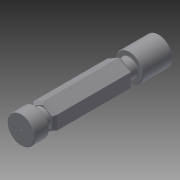
# Autodesk Inventor part: Part1
Saved by Autodesk Inventor 2015 SP2 (Build 190223200, 223)
## iProperties
Created: 2015-11-09
Part Number: Part1
Material: Generic
Document SubType Name: Modeling
Designer: KC-019
Density: 1 g/cm^3
Appearance: Default
Author: KC-019
Autodesk Inventor part; units mm, degrees
ref_plane "YZ Plane" through (0, 0, 0) normal (1, 0, 0) x (0, 1, 0)
ref_plane "XZ Plane" through (0, 0, 0) normal (0, 1, 0) x (-1, 0, 0)
ref_plane "XY Plane" through (0, 0, 0) normal (0, 0, 1) x (1, 0, 0)
sketch "Sketch1" plane through (0, 0, 0) normal (0, 0, 1) x (1, 0, 0)
  circle A0 centre (0, 0) radius 17.6911
  dimension "d0" = 35.3822
  constraints: 1 centre point, 1 coincident
  measures "d0" diameter of A0
extrude "Extrusion1" add sketch "Sketch1" along normal blind 38.1
sketch "Sketch2" plane through (0, 0, 38.1) normal (0, 0, 1) x (1, 0, 0)
  circle A0 centre (0, 0) radius 11.2776
  dimension "d3" = 22.5552
  constraints: 1 centre point, 1 coincident
  measures "d3" diameter of A0
extrude "Extrusion2" add sketch "Sketch2" along normal blind 9.9314
sketch "Sketch4" plane through (0, 0, 48.0314) normal (0, 0, 1) x (1, 0, 0)
  line L0 (0, 17.4198) -> (15.086, 8.7099)
  line L1 (15.086, 8.7099) -> (15.086, -8.7099)
  line L2 (15.086, -8.7099) -> (0, -17.4198)
  line L3 (0, -17.4198) -> (-15.086, -8.7099)
  line L4 (-15.086, -8.7099) -> (-15.086, 8.7099)
  line L5 (-15.086, 8.7099) -> (0, 17.4198)
  point P0 (0, 0)
  point P1 (0, 0)
  constraints: 12 end point, 1 coincident, 13 other
extrude "Extrusion4" add sketch "Sketch4" along normal blind 100.838
sketch "Sketch5" plane through (0, 0, 148.8694) normal (0, 0, 1) x (1, 0, 0)
  circle A0 centre (0, 0) radius 11.2776
  constraints: 1 centre point, 1 coincident
extrude "Extrusion5" add sketch "Sketch5" along normal blind 9.2202
sketch "Sketch6" plane through (0, 0, 158.0896) normal (0, 0, 1) x (1, 0, 0)
  circle A0 centre (0, 0) radius 17.6911
  constraints: 1 centre point, 1 coincident
extrude "Extrusion6" add sketch "Sketch6" along normal blind 18.542
fillet "Fillet1" radius 1.016 1 edges at (-17.6911, 0, 176.6316)
fillet "Fillet2" radius 0.889 1 edges at (-11.2776, 0, 158.0896)
chamfer "Chamfer1" distance 3.175 angle 45 12 edges at (7.543, 13.0648, 148.8694) (15.086, 0, 148.8694) (7.543, -13.0648, 148.8694) (-7.543, -13.0648, 148.8694) (-15.086, 0, 148.8694) (-7.543, 13.0648, 148.8694) (-7.543, -13.0648, 48.0314) (-15.086, 0, 48.0314) (7.543, -13.0648, 48.0314) (15.086, 0, 48.0314) (-7.543, 13.0648, 48.0314) (7.543, 13.0648, 48.0314)
fillet "Fillet3" radius 0.889 1 edges at (-11.2776, 0, 38.1)
fillet "Fillet4" radius 1.016 1 edges at (-17.6911, 0, 0)
fillet "Fillet5" radius 1.016 1 edges at (-17.6911, 0, 38.1)
fillet "Fillet6" radius 1.016 1 edges at (-17.6911, 0, 158.0896)
sketch "Sketch7" plane through (0, 0, 176.6316) normal (0, 0, 1) x (1, 0, 0)
  circle A0 centre (0, 0) radius 11.2776 projected
  circle A1 centre (0, 0) radius 0.9525
  dimension "d23" = 1.905
  constraints: 1 centre point, 1 coincident
  measures "d23" diameter of A1
extrude "Extrusion7" cut sketch "Sketch7" against normal blind 5.08 contours A1
sketch "Sketch8" plane through (0, 0, 0) normal (0, 0, -1) x (-1, 0, 0)
  circle A0 centre (0, 0) radius 0.9525 projected
  circle A1 centre (0, 0) radius 0.9525
  constraints: 1 centre point, 1 coincident
extrude "Extrusion8" cut sketch "Sketch8" against normal blind 5.08
body "Solid1"
